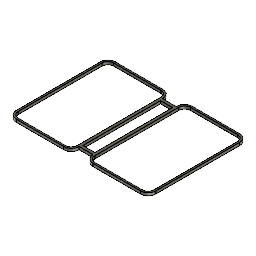
footpedal (Autodesk Fusion 360 design; units mm, degrees)
Autodesk Fusion 360 part; units mm, degrees
sketch "Sketch1" plane through (0, 0, 0) normal (0, 0, 1) x (1, 0, 0)
  line L0 (-27.3219, 46.2488) -> (22.1781, 46.2488)
  line L1 (28.1781, 40.2488) -> (28.1781, -47.2512)
  line L2 (22.1781, -53.2512) -> (-27.3219, -53.2512)
  line L3 (-33.3219, -47.2512) -> (-33.3219, 40.2488)
  arc A0 (28.1781, 40.2488) -> (22.1781, 46.2488) centre (22.1781, 40.2488) ccw
  arc A1 (-33.3219, -47.2512) -> (-27.3219, -53.2512) centre (-27.3219, -47.2512) ccw
  arc A2 (22.1781, -53.2512) -> (28.1781, -47.2512) centre (22.1781, -47.2512) ccw
  arc A3 (-27.3219, 46.2488) -> (-33.3219, 40.2488) centre (-27.3219, 40.2488) ccw
  arc A4 (22.1781, -55.2512) -> (30.1781, -47.2512) centre (22.1781, -47.2512) ccw
  line L4 (30.1781, 40.2488) -> (30.1781, -47.2512)
  arc A5 (30.1781, 40.2488) -> (22.1781, 48.2488) centre (22.1781, 40.2488) ccw
  line L5 (-27.3219, 48.2488) -> (22.1781, 48.2488)
  arc A6 (-27.3219, 48.2488) -> (-35.3219, 40.2488) centre (-27.3219, 40.2488) ccw
  line L6 (-35.3219, -47.2512) -> (-35.3219, 40.2488)
  arc A7 (-35.3219, -47.2512) -> (-27.3219, -55.2512) centre (-27.3219, -47.2512) ccw
  line L7 (22.1781, -55.2512) -> (-27.3219, -55.2512)
  line L8 (52.6781, 48.2488) -> (102.1781, 48.2488)
  line L9 (102.1781, -55.2512) -> (52.6781, -55.2512)
  line L10 (102.1781, -53.2512) -> (52.6781, -53.2512)
  arc A8 (102.1781, -53.2512) -> (108.1781, -47.2512) centre (102.1781, -47.2512) ccw
  line L11 (110.1781, 40.2488) -> (110.1781, -47.2512)
  arc A9 (46.6781, -47.2512) -> (52.6781, -53.2512) centre (52.6781, -47.2512) ccw
  line L12 (46.6781, -47.2512) -> (46.6781, 40.2488)
  line L13 (44.6781, -47.2512) -> (44.6781, 40.2488)
  arc A10 (108.1781, 40.2488) -> (102.1781, 46.2488) centre (102.1781, 40.2488) ccw
  arc A11 (52.6781, 46.2488) -> (46.6781, 40.2488) centre (52.6781, 40.2488) ccw
  arc A12 (52.6781, 48.2488) -> (44.6781, 40.2488) centre (52.6781, 40.2488) ccw
  arc A13 (44.6781, -47.2512) -> (52.6781, -55.2512) centre (52.6781, -47.2512) ccw
  arc A14 (102.1781, -55.2512) -> (110.1781, -47.2512) centre (102.1781, -47.2512) ccw
  arc A15 (110.1781, 40.2488) -> (102.1781, 48.2488) centre (102.1781, 40.2488) ccw
  line L14 (52.6781, 46.2488) -> (102.1781, 46.2488)
  line L15 (108.1781, 40.2488) -> (108.1781, -47.2512)
  line L16 (44.6781, 39.6601) -> (44.6781, -47.2512)
  line L17 (30.1781, -47.2512) -> (30.1781, 39.6601)
  line L18 (28.1781, 39.6696) -> (46.6781, 39.6696)
  line L19 (46.6781, 39.6696) -> (46.6781, -47.2512)
  line L20 (46.6781, -47.2512) -> (28.1781, -47.2512)
  line L21 (28.1781, -47.2512) -> (28.1781, 39.6696)
  line L22 (43.6781, -44.2512) -> (31.1781, -44.2512)
  line L23 (31.1781, -44.2512) -> (31.1781, 36.6696)
  line L24 (31.1781, 36.6696) -> (43.6781, 36.6696)
  line L25 (43.6781, 36.6696) -> (43.6781, -44.2512)
  point P0 (-33.3219, 46.2488)
  point P1 (28.1781, 46.2488)
  point P2 (-33.3219, -53.2512)
  point P3 (108.1781, 46.2488)
  point P4 (46.6781, -53.2512)
  point P5 (46.6781, 46.2488)
  point P6 (80, 0)
  dimension "d1" = 61.5
  dimension "d2" = 99.5
  dimension "d3" = 6
  dimension "d4" = 2
  dimension "d7" = 80
  dimension "d8" = 0
  dimension "d11" = 3
  measures "d1" distance of P0 P1
  measures "d2" distance of P0 P2
  measures "d3" radius of A0
extrude "Extrude1" add sketch "Sketch1" along normal blind 3 contours L0 L1 L2 L3 A0 A1 A2 A3 A4 L4 A5 L5 A6 L6 A7 L7 L18 L20 | L1 L4 L17 L18 L20 L21 | L4 L13 L16 L17 L18 L20 | L12 L13 L16 L18 L19 L20 | L8 L9 L10 A8 L11 A9 L12 L13 A10 A11 A12 A13 A14 A15 L14 L15 L18 L20
